PLATE_LV_TOP (Autodesk Fusion 360 design; units mm, degrees)
Autodesk Fusion 360 part; units mm, degrees
note: some values were not read from the file. Set by a fixed rule: which sketch regions a step uses.
sketch "Esquisse1" plane through (0, 0, 0) normal (0, 0, 1) x (1, 0, 0)
  line L0 (100, 78) -> (-100, 78)
  line L1 (-100, 78) -> (-100, -78)
  line L2 (-100, -78) -> (100, -78)
  line L3 (100, -78) -> (100, 78)
  line L4 (100, 78) -> (-100, -78) construction
  line L5 (-100, 78) -> (100, -78) construction
  line L6 (103, -75) -> (-103, -75)
  line L7 (-103, -75) -> (-103, 75)
  line L8 (-103, 75) -> (103, 75)
  line L9 (103, 75) -> (103, -75)
  line L10 (103, -75) -> (-103, 75) construction
  line L11 (-103, -75) -> (103, 75) construction
  dimension "d1" = 200
  dimension "d2" = 206
  dimension "d3" = 150
  dimension "d4" = 156
  constraint horizontal L0
  constraint perpendicular L0 L1
  constraint parallel L0 L2
  constraint parallel L1 L3
  constraint coincident L4 origin
  constraint coincident L5 origin
  constraint horizontal L6
  constraint perpendicular L6 L7
  constraint parallel L6 L8
  constraint parallel L7 L9
  constraint coincident L10 origin
  constraint coincident L11 origin
  measures "d1" distance of L0.start L0.end
  measures "d2" distance of L7.end L8.end
  measures "d3" distance of L6.end L7.end
  measures "d4" distance of L0.end L1.end
extrude "Extrusion1" add sketch "Esquisse1" along normal blind 3
sketch "Esquisse4" plane through (0, 0, 3) normal (0, 0, 1) x (-1, 0, 0)
  line L0 (-100, -75) -> (-100, -78)
  line L1 (-100, -78) -> (100, -78)
  line L2 (100, -78) -> (100, -75)
  line L3 (100, -75) -> (103, -75)
  line L4 (103, -75) -> (103, 75)
  line L5 (103, 75) -> (100, 75)
  line L6 (100, 75) -> (100, 78)
  line L7 (100, 78) -> (-100, 78)
  line L8 (-100, 78) -> (-100, 75)
  line L9 (-100, 75) -> (-103, 75)
  line L10 (-103, 75) -> (-103, -75)
  line L11 (-103, -75) -> (-100, -75)
  line L12 (-2.5, 49) -> (67, 49)
  line L13 (67, 49) -> (67, -49)
  line L14 (67, -49) -> (-2.5, -49)
  line L15 (-2.5, -49) -> (-2.5, 49)
  line L16 (-2.5, 49) -> (67, -49) construction
  line L17 (67, 49) -> (-2.5, -49) construction
  line L18 (-48, 48) -> (-20.5, 48)
  line L19 (-20.5, 48) -> (-20.5, -27)
  line L20 (-20.5, -27) -> (-48, -27)
  line L21 (-48, -27) -> (-48, 48)
  line L22 (-48, 48) -> (-20.5, -27) construction
  line L23 (-20.5, 48) -> (-48, -27) construction
  circle A0 centre (67, -49) radius 1.7
  circle A1 centre (-2.5, -49) radius 1.7
  circle A2 centre (-20.5, -27) radius 1.6
  circle A3 centre (-48, -27) radius 1.6
  circle A4 centre (-20.5, 48) radius 1.6
  circle A5 centre (-48, 48) radius 1.6
  line L24 (67, -49) -> (-2.5, -49)
  line L25 (-2.5, -49) -> (-2.5, 38)
  line L26 (-2.5, 38) -> (67, 38)
  line L27 (67, 38) -> (67, -49)
  circle A6 centre (67, 49) radius 1.7
  circle A7 centre (-2.5, 38) radius 1.7
  line L28 (-83, -15) -> (-83, 15)
  line L29 (-68, -20) -> (-78, -20)
  arc A8 (-68, -20) -> (-63, -15) centre (-68, -15) ccw
  line L30 (-63, 20) -> (-83, -20) construction
  line L31 (-78, 20) -> (-68, 20)
  arc A9 (-63, 15) -> (-68, 20) centre (-68, 15) ccw
  arc A10 (-78, 20) -> (-83, 15) centre (-78, 15) ccw
  line L32 (-83, 20) -> (-63, -20) construction
  line L33 (-63, 15) -> (-63, -15)
  arc A11 (-83, -15) -> (-78, -20) centre (-78, -15) ccw
  point P0 (32.25, 0)
  point P1 (-34.25, 10.5)
  point P2 (-73, 0)
  dimension "d26" = 69.5
  dimension "d27" = 98
  dimension "d28" = 27.5
  dimension "d29" = 75
  dimension "d30" = 18
  dimension "d31" = 3.4
  dimension "d34" = 3.4
  dimension "d35" = 3.2
  dimension "d36" = 3.2
  dimension "d37" = 3.2
  dimension "d38" = 3.2
  dimension "d39" = 87
  dimension "d43" = 3.4
  dimension "d44" = 3.4
  dimension "d45" = 5
  dimension "d46" = 20
  dimension "d47" = 15
  dimension "d48" = 20
  dimension "d49" = 40
  dimension "d50" = 29
  dimension "d51" = 58
  dimension "d52" = 30
  constraint horizontal L12
  constraint perpendicular L12 L13
  constraint parallel L12 L14
  constraint parallel L13 L15
  constraint coincident L16 P0
  constraint coincident L17 P0
  constraint horizontal L18
  constraint perpendicular L18 L19
  constraint parallel L18 L20
  constraint parallel L19 L21
  constraint coincident L22 P1
  constraint coincident L23 P1
  constraint coincident L13.end L14.start
  constraint coincident L14.end L15.start
  constraint coincident L19.end L20.start
  constraint coincident L20.end L21.start
  constraint coincident L18.end L19.start
  constraint coincident L18.start L21.end
  constraint horizontal L24
  constraint vertical L25
  constraint horizontal L26
  constraint vertical L27
  constraint coincident L15 L25.end
  constraint coincident L12.end L13.start
  constraint coincident L25.end L26.start
  constraint horizontal L31
  constraint perpendicular L31 L33
  constraint parallel L29 L31
  constraint parallel L28 L33
  constraint coincident P2 L32
  constraint coincident P2 L30
  constraint coincident L32.end L33
  constraint coincident L32.end L29
  constraint tangent A8 L33
  constraint tangent L29 A8
  constraint coincident L30.end L28
  constraint coincident L30.end L29
  constraint tangent L28 A11
  constraint tangent L29 A11
  constraint equal A8 A11
  constraint coincident L32.start L28
  constraint coincident L32.start L31
  constraint tangent L28 A10
  constraint tangent L31 A10
  constraint equal A8 A10
  constraint coincident L30.start L31
  constraint coincident L30.start L33
  constraint tangent L31 A9
  constraint tangent A9 L33
  constraint equal A8 A9
  measures "d26" distance of L13.end L14.end
  measures "d27" distance of L12.end L13.end
  measures "d28" distance of L19.end L20.end
  measures "d29" distance of L18.end L19.end
  measures "d30" distance of L15 L19
  measures "d31" diameter of A0
  measures "d34" diameter of A1
  measures "d35" diameter of A2
  measures "d36" diameter of A3
  measures "d37" diameter of A4
  measures "d38" diameter of A5
  measures "d39" distance of L13.end L26.end
  measures "d43" diameter of A6
  measures "d44" diameter of A7
  measures "d45" radius of A8
  measures "d46" distance of L10 L28
  measures "d47" distance of L21 L33
  measures "d48" distance of L28 L33
  measures "d49" distance of L29 L31
  measures "d50" distance of L7 L12
  measures "d51" distance of L7 L31
  measures "d52" distance of L7 L18
extrude "Extrusion4" cut sketch "Esquisse4" against normal blind 3 contours L12 L13 A6 | L12 L13 A6 | L15 L26 A7 | L15 L25 A7 | L15 L25 L26 A7 | L14 L15 A1 L24 L25 | L14 L15 A1 L24 L25 | L13 L14 A0 L24 L27 | L13 L14 A0 L24 L27 | L18 L21 A5 | L18 L21 A5 | L18 L19 A4 | L18 L19 A4 | L20 L21 A3 | L20 L21 A3 | L19 L20 A2 | L19 L20 A2 | L28 L29 A8 L31 A9 A10 L33 A11
equation "d2 = d1 + ( 2 * 3 ) * 1 mm"
equation "d4 = d3 + ( 2 * 3 ) * 1 mm"
